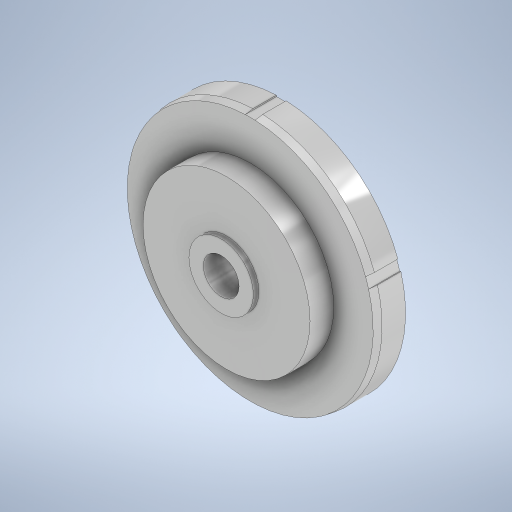
# Autodesk Inventor part: main_motor_planet
Saved by Autodesk Inventor 2023 (Build 270158000, 158)
## iProperties
Created: 2023-11-23
Part Number: main_motor_planet
Material: Aluminum 6061-AHC
Document SubType Name: Modeling
Designer: aaron
Density: 2.7 g/cm^3
Appearance: Aluminum - Dark
Author: aaron
Autodesk Inventor part; units mm, degrees
ref_plane "YZ Plane" through (0, 0, 0) normal (1, 0, 0) x (0, 1, 0)
ref_plane "XZ Plane" through (0, 0, 0) normal (0, 1, 0) x (-1, 0, 0)
ref_plane "XY Plane" through (0, 0, 0) normal (0, 0, 1) x (1, 0, 0)
sketch "Sketch1" plane through (0, 0, 0) normal (0, 0, 1) x (1, 0, 0)
  circle A0 centre (0, 0) radius 52.025
  line L0 (-2.05, 56.1236) -> (2.05, 56.1236)
  line L1 (2.05, 56.1236) -> (2.05, 48.6562)
  line L2 (2.05, 48.6562) -> (-2.05, 48.6562)
  line L3 (-2.05, 48.6562) -> (-2.05, 56.1236)
  line L4 (0, 0) -> (0, 78.5962)
  circle A1 centre (0, 0) radius 51.475
  line L5 (-54.0102, 15.3935) -> (-52.7433, 19.2928)
  line L6 (-52.7433, 19.2928) -> (-45.6413, 16.9853)
  line L7 (-45.6413, 16.9853) -> (-46.9083, 13.0859)
  line L8 (-46.9083, 13.0859) -> (-54.0102, 15.3935)
  line L9 (-31.3302, -46.6099) -> (-34.6471, -44.2)
  line L10 (-34.6471, -44.2) -> (-30.2579, -38.1587)
  line L11 (-30.2579, -38.1587) -> (-26.9409, -40.5687)
  line L12 (-26.9409, -40.5687) -> (-31.3302, -46.6099)
  line L13 (34.6471, -44.2) -> (31.3302, -46.6099)
  line L14 (31.3302, -46.6099) -> (26.9409, -40.5687)
  line L15 (26.9409, -40.5687) -> (30.2579, -38.1587)
  line L16 (30.2579, -38.1587) -> (34.6471, -44.2)
  line L17 (52.7433, 19.2928) -> (54.0102, 15.3935)
  line L18 (54.0102, 15.3935) -> (46.9083, 13.0859)
  line L19 (46.9083, 13.0859) -> (45.6413, 16.9853)
  line L20 (45.6413, 16.9853) -> (52.7433, 19.2928)
  point P0 (2.05, 51.4342)
  point P1 (-2.05, 51.4342)
  point P2 (-2.05, 51.9846)
  point P3 (-48.8068, 18.0138)
  point P4 (-48.2833, 17.8437)
  point P5 (-49.5503, 13.9444)
  point P6 (-50.0738, 14.1145)
  point P7 (-32.2143, -40.8515)
  point P8 (-31.8907, -40.4062)
  point P9 (-28.5738, -42.8161)
  point P10 (-28.8973, -43.2614)
  point P11 (28.8973, -43.2614)
  point P12 (28.5738, -42.8161)
  point P13 (31.8907, -40.4062)
  point P14 (32.2143, -40.8515)
  point P15 (50.0738, 14.1145)
  point P16 (49.5503, 13.9444)
  point P17 (48.2833, 17.8437)
  point P18 (48.8068, 18.0138)
  point P19 (2.05, 51.9846)
  dimension "d0" = 104.05
  dimension "d2" = 0.55
  dimension "d3" = 2.05
  dimension "d4" = 4.1
  dimension "d7" = 360
  constraints: 42 end point, 2 centre point, 2 parallel, 1 coincident, 1 horizontal, 1 perpendicular, 1 vertical, 41 other
  measures "d0" diameter of A0
  measures "d2" radial gap between concentric circles of A0 A1
  measures "d3" distance between parallel lines of L1 L4
  measures "d4" distance of L0.start L0.end
extrude "Extrusion1" add sketch "Sketch1" along normal blind 13 contours A0 L16 A1 L18 | L20 A1 L1 A0 | L18 L19 L20 A1 | A1 L16 L15 L14 L12 L11 L10 L8 L7 L6 L3 L2 L1 L20 L19 L18 | A0 L12 A1 L14 | A1 L14 L15 L16 | L1 L2 L4 A1 | A0 L8 A1 L10 | A1 L10 L11 L12 | L3 A1 L6 A0 | L4 L2 L3 A1 | A1 L6 L7 L8
chamfer "Chamfer1" distance 0.55 distance2 3.2 5 edges at (49.4787, -16.0766, 13) (0, -52.025, 13) (-49.4787, -16.0766, 13) (-30.5795, 42.0891, 13) (30.5795, 42.0891, 13) measured on face at (-10.4211, -2.2799, 13)
sketch "Sketch2" plane through (0, 0, 0) normal (0, 0, -1) x (-1, 0, 0)
  circle A0 centre (0, 0) radius 22
  dimension "d14" = 44
  constraints: 1 centre point, 1 coincident
  measures "d14" diameter of A0
extrude "Extrusion2" add sketch "Sketch2" along normal blind 4
sketch "Sketch3" plane through (0, 0, 13) normal (0, 0, 1) x (1, 0, 0)
  circle A0 centre (0, 0) radius 34.95
  dimension "d17" = 69.9
  constraints: 1 centre point, 1 coincident
  measures "d17" diameter of A0
extrude "Extrusion3" add sketch "Sketch3" along normal blind 9.9
sketch "Sketch4" plane through (0, 0, 22.9) normal (0, 0, 1) x (1, 0, 0)
  circle A0 centre (0, 0) radius 13.5
  dimension "d20" = 27
  constraints: 1 centre point, 1 coincident
  measures "d20" diameter of A0
extrude "Extrusion4" add sketch "Sketch4" along normal blind 2.25
sketch "Sketch5" plane through (0, 0, 25.15) normal (0, 0, 1) x (1, 0, 0)
  circle A0 centre (0, 0) radius 7.5
  dimension "d23" = 15
  constraints: 1 centre point, 1 coincident
  measures "d23" diameter of A0
extrude "Extrusion5" cut sketch "Sketch5" against normal through all
body "Solid1"
